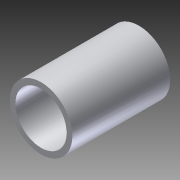
# Autodesk Inventor part: V5 Shooter Conveyor Roller
Saved by Autodesk Inventor 2014 SP1 (Build 180222100, 222)
## iProperties
Created: 2012-02-10
Part Number: V5 Shooter Conveyor Roller
Material: PVC-Piping
Document SubType Name: Modeling
Designer: Moses
Mass: 42.4444 g
Surface Area: 168.328 cm^2
Volume: 30.3174 cm^3
Density: 1.4 g/cm^3
Appearance: Smooth - White
Author: Moses
Autodesk Inventor part; units mm, degrees
ref_plane "YZ Plane" through (0, 0, 0) normal (1, 0, 0) x (0, 1, 0)
ref_plane "XZ Plane" through (0, 0, 0) normal (0, 1, 0) x (-1, 0, 0)
ref_plane "XY Plane" through (0, 0, 0) normal (0, 0, 1) x (1, 0, 0)
sketch "Sketch1" plane through (0, 0, 0) normal (0, 0, 1) x (1, 0, 0)
  circle A0 centre (0, 0) radius 17.272
  circle A1 centre (0, 0) radius 21.082
  dimension "d0" = 34.544
  dimension "d1" = 42.164
  constraints: 2 centre point, 2 coincident
  measures "d0" diameter of A0
  measures "d1" diameter of A1
extrude "Extrusion1" add sketch "Sketch1" along normal blind 66.04
body "Solid1"
